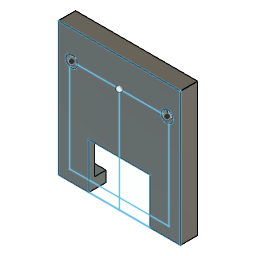
placa_cima (Autodesk Fusion 360 design; units mm, degrees)
part number: 2025-10-18-19-38-59-563
Autodesk Fusion 360 part; units mm, degrees
sketch "Sketch3" plane through (0, 0, 0) normal (0, 1, 0) x (1, 0, 0)
  line L0 (11, 2.882) -> (-21, 2.882)
  line L1 (-21, 2.882) -> (-21, -32.118)
  line L2 (-21, -32.118) -> (11, -32.118)
  line L3 (11, -32.118) -> (11, 2.882)
  line L4 (-5, -24.618) -> (-5, 2.882)
  circle A0 centre (-17.5, -24.618) radius 1.5
  circle A1 centre (7.5, -24.618) radius 1.5
  line L5 (-17.5, -24.618) -> (7.5, -24.618)
  line L6 (-5, 0.0503) -> (-18, 0.0503)
  line L7 (-5, 0.0503) -> (8, 0.0503)
  line L8 (-18, 0.0503) -> (-18, -23.2038)
  line L9 (8, 0.0503) -> (8, -23.2038)
  line L10 (-5, 2.882) -> (-13, 2.882)
  line L11 (-5, 2.882) -> (3, 2.882)
  line L12 (-13, 2.882) -> (-13, -9.118)
  line L13 (3, 2.882) -> (3, -9.118)
  line L14 (-13, -9.118) -> (3, -9.118)
  dimension "d32" = 35
  dimension "d33" = 32
  dimension "d58" = 27.5
  dimension "d61" = 3
  dimension "d62" = 3
  dimension "d63" = 13
  dimension "d64" = 13
  dimension "d66" = 8
  dimension "d67" = 8
  dimension "d68" = 12
  dimension "d69" = 12
  dimension "d70" = 16
  dimension "d71" = 23.2541
  constraint horizontal L0
  constraint vertical L1
  constraint horizontal L2
  constraint vertical L3
  constraint midpoint L0 L4.end
  constraint coincident A0.centre L5.start
  constraint coincident A1.centre L5.end
  constraint coincident L4 L6.start
  constraint perpendicular L4 L6
  constraint perpendicular L4 L7
  constraint coincident A0 L8.end
  constraint perpendicular L6 L8
  constraint coincident A1 L9.end
  constraint perpendicular L7 L9
  constraint coincident L0 L10.end
  constraint coincident L0 L11.end
  constraint perpendicular L6 L12
  constraint perpendicular L11 L13
  measures "d32" distance of L0.start L2.end
  measures "d33" distance of L0.start L0.end
  measures "d58" distance of L4.end L4.start
  measures "d61" diameter of A0
  measures "d62" diameter of A1
  measures "d63" distance of L6.start L6.end
  measures "d64" distance of L6.start L7.end
  measures "d66" distance of L4.end L10.end
  measures "d67" distance of L4.end L11.end
  measures "d68" distance of L10.end L12.end
  measures "d69" distance of L11.end L13.end
  measures "d70" distance of L12.end L13.end
  measures "d71" distance of L6.end L8.end
extrude "Extrude7" add sketch "Sketch3" along normal blind 4.5 contours L0 L1 L2 L3 A0 A1 L5 L6 L7 L8 L9 L12 L13
extrude "Extrude8" add sketch "Sketch3" along normal blind 1.5 contours L4 A1 L5 L7 L9 L13 L14 | L4 A0 L5 L6 L8 L12 L14
